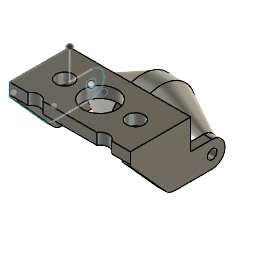
Robot Chassis Version 2 (Autodesk Fusion 360 archive; units mm, degrees)
design "Guide wheel base"
part number: 2026-03-02-16-28-39-596
Autodesk Fusion 360 part; units mm, degrees
sketch "Sketch1" plane through (0, 0, 0) normal (0, 0, 1) x (1, 0, 0)
  line L0 (14.05, 32) -> (-14.05, 32)
  line L1 (-14.05, 32) -> (-14.05, 18)
  line L2 (-14.05, 18) -> (14.05, 18)
  line L3 (14.05, 18) -> (14.05, 32)
  line L4 (14.05, 32) -> (-14.05, 18) construction
  line L5 (-14.05, 32) -> (14.05, 18) construction
  circle A0 centre (0, 25) radius 4
  line L6 (-4, 25) -> (-6.2, 25)
  line L7 (4, 25) -> (6.2, 25)
  circle A1 centre (-8.2, 25) radius 2
  circle A2 centre (8.2, 25) radius 2
  circle A3 centre (-8, 17) radius 2
  circle A4 centre (8, 17) radius 2
  point P0 (0, 25)
  dimension "d1" = 28.1
  dimension "d2" = 14
  dimension "d3" = 8
  dimension "d4" = 2.2
  dimension "d5" = 2.2
  dimension "d6" = 4
  dimension "d7" = 4
  dimension "d8" = 4
  dimension "d9" = 4
  constraint horizontal L0
  constraint perpendicular L0 L1
  constraint parallel L0 L2
  constraint parallel L1 L3
  constraint coincident L4 P0
  constraint coincident L5 P0
  constraint coincident P0 A0.centre
  constraint coincident A0 L6.start
  constraint horizontal L6
  constraint coincident A0 L7.start
  constraint horizontal L7
  constraint coincident L6.end A1
  constraint coincident L7.end A2
  measures "d1" distance of L1.end L2.end
  measures "d2" distance of L0.end L1.end
  measures "d3" diameter of A0
  measures "d4" distance of L6.start L6.end
  measures "d5" distance of L7.start L7.end
  measures "d6" diameter of A1
  measures "d7" diameter of A2
  measures "d8" diameter of A3
  measures "d9" diameter of A4
extrude "Extrude1" add sketch "Sketch1" along normal blind 2 contours L0 L1 L2 L3 A3 A4 makes body 1
move_body "Move1" bodies 1 to x (1, 0, 0) y (0, 1, 0) z (0, 0, 1) at (0, 0, 15)
sketch "Sketch2" plane through (-14.05, 0, 0) normal (-1, 0, 0) x (0, -1, 0)
  line L0 (-32, 15) -> (-18, 15)
  line L1 (-18, 15) -> (-18, 17)
  line L2 (-18, 17) -> (-32, 17)
  line L3 (-32, 17) -> (-32, 15)
  line L4 (-32, 17) -> (-18, 17)
  line L5 (-28.3361, 4) -> (-32, 4)
  line L6 (-32, 4) -> (-37, 4)
  line L7 (-37, 10) -> (-32, 10)
  line L8 (-18.2567, 13.7148) -> (-26.1062, 4.9931)
  arc A0 (-37, 10) -> (-40, 7) centre (-37, 7) ccw
  arc A1 (-40, 7) -> (-37, 4) centre (-37, 7) ccw
  arc A2 (-28.3361, 4) -> (-26.1062, 4.9931) centre (-28.3361, 7) ccw
  line L9 (-18, 17) -> (-18, 14.3837)
  line L10 (-32, 17) -> (-32, 10)
  arc A3 (-18.2567, 13.7148) -> (-18, 14.3837) centre (-19, 14.3837) ccw
  circle A4 centre (-37, 7) radius 1.1
  point P0 (-40, 4)
  dimension "d12" = 13
  dimension "d13" = 8
  dimension "d14" = 6
  dimension "d15" = 3
  dimension "d16" = 3
  dimension "d17" = 3
  dimension "d18" = 1
  dimension "d25" = 2.2
  constraint horizontal L4
  constraint horizontal L5
  constraint coincident L2.end L3.start
  constraint horizontal L6
  constraint horizontal L7
  constraint tangent L7 A0
  constraint coincident P0 L6
  constraint tangent L6 A1
  constraint coincident A0.end A1.start
  constraint tangent L8 A2
  constraint tangent L5 A2
  constraint perpendicular L4 L9
  constraint perpendicular L7 L10
  constraint tangent L8 A3
  constraint tangent L9 A3
  constraint concentric A0 A4
  measures "d12" distance of L2.end L5.end
  measures "d13" distance of L5.end P0
  measures "d14" distance of L5.end L7.end
  measures "d15" radius of A0
  measures "d16" radius of A1
  measures "d17" radius of A2
  measures "d18" radius of A3
  measures "d25" diameter of A4
extrude "Extrude2" add sketch "Sketch2" against normal blind 28.1 contours L0 L5 L6 L7 L8 A0 A1 A2 L9 L10 A3 | A4 bodies 1
sketch "Sketch3" plane through (0, 16.9061, 15.2155) normal (0, -0.743294, -0.668965) x (1, 0, 0)
  line L0 (-14.05, -2.019) -> (-14.05, -13.7528)
  line L1 (-14.05, -13.7528) -> (14.05, -13.7528)
  line L2 (14.05, -13.7528) -> (14.05, -2.019)
  line L3 (14.05, -2.019) -> (-14.05, -2.019)
sketch "Sketch4" plane through (0, 18, 0) normal (0, -1, 0) x (1, 0, 0)
  line L0 (14.05, 14.3837) -> (14.05, 17)
  line L1 (-9.7321, 17) -> (-14.05, 17)
  line L2 (-14.05, 17) -> (-14.05, 14.3837)
  line L3 (-14.05, 14.3837) -> (14.05, 14.3837)
  line L4 (-14.05, 4.9931) -> (-14.05, 4)
  line L5 (-14.05, 4) -> (14.05, 4)
  line L6 (14.05, 4) -> (14.05, 4.9931)
  line L7 (14.05, 4.9931) -> (-14.05, 4.9931)
  line L8 (-14.05, 14.3837) -> (-14.05, 13.7148)
  line L9 (-14.05, 13.7148) -> (14.05, 13.7148)
  line L10 (14.05, 13.7148) -> (14.05, 14.3837)
  line L11 (14.05, 14.3837) -> (-14.05, 14.3837)
  line L12 (-14.05, 13.7148) -> (-14.05, 4.9931)
  line L13 (-14.05, 4.9931) -> (14.05, 4.9931)
  line L14 (14.05, 4.9931) -> (14.05, 13.7148)
  line L15 (14.05, 13.7148) -> (-14.05, 13.7148)
  line L16 (-14.05, 14.3837) -> (-12.05, 14.3837)
  line L17 (-12.05, 14.3837) -> (-12.05, 4)
  line L18 (-12.05, 4) -> (-14.05, 4)
  line L19 (-14.05, 4) -> (-14.05, 14.3837)
  line L20 (14.05, 14.3837) -> (12.05, 14.3837)
  line L21 (12.05, 14.3837) -> (12.05, 4)
  line L22 (12.05, 4) -> (14.05, 4)
  line L23 (14.05, 4) -> (14.05, 14.3837)
  line L24 (-9.7321, 15) -> (-9.7321, 17)
  line L25 (14.05, 17) -> (9.7321, 17)
  line L26 (9.7321, 17) -> (9.7321, 15)
  line L27 (9.7321, 15) -> (6.2679, 15)
  line L28 (6.2679, 15) -> (6.2679, 17)
  line L29 (6.2679, 17) -> (-6.2679, 17)
  line L30 (-6.2679, 17) -> (-6.2679, 15)
  line L31 (-6.2679, 15) -> (-9.7321, 15)
  dimension "d21" = 2
  dimension "d22" = 2
  constraint horizontal L16
  constraint vertical L17
  constraint horizontal L18
  constraint vertical L19
  constraint coincident L5 L17.end
  constraint coincident L2.end L3.start
  constraint horizontal L20
  constraint vertical L21
  constraint horizontal L22
  constraint vertical L23
  constraint coincident L0.start L3.end
  measures "d21" distance of L2.end L16.end
  measures "d22" distance of L0.start L20.end
extrude "Extrude3" cut sketch "Sketch4" against normal blind 25.5 contours L3 L9 L11 L15 L17 L21 | L7 L9 L13 L15 L17 L21 | L5 L7 L13 L17 L21 bodies 1
delete_face "DeleteFace1" 2 faces at (-7.8346, 18.4227, 15) (8.2893, 18.432, 15) on bodies 1
delete_face "DeleteFace2" 3 faces at (-8.0517, 24.35, 15) (1.6687, 25.926, 15) (7.5851, 25.0994, 15) on bodies 1
extrude "Extrude4" cut sketch "Sketch2" against normal blind 33 contours A4 bodies 1
sketch "Sketch5" plane through (0, 0, 0) normal (0, 1, 0) x (1, 0, 0)
  line L0 (12, -7, 37) -> (-12, -7, 37)
  line L1 (-2.2, 1, 37) -> (2.2, 1, 37)
  line L2 (2.2, 1, 37) -> (2.2, -15, 37)
  line L3 (2.2, -15, 37) -> (-2.2, -15, 37)
  line L4 (-2.2, -15, 37) -> (-2.2, 1, 37)
  line L5 (-2.2, 1, 37) -> (2.2, -15, 37) construction
  line L6 (2.2, 1, 37) -> (-2.2, -15, 37) construction
  line L7 (12, -10, 37) -> (12, -4, 37)
  line L8 (12, -4, 37) -> (2.2, 1, 37)
  line L9 (-12, -10, 37) -> (-12, -4, 37)
  line L10 (-12, -4, 37) -> (-2.2, 1, 37)
  line L11 (12, -10, 37) -> (2.2, -15, 37)
  line L12 (-2.2, -15, 37) -> (-12, -10, 37)
  point P0 (0, -7)
  dimension "d28" = 4.4
  dimension "d29" = 16
revolve "Revolve1" add sketch "Sketch5" angle 360 about axis through (12, 37, 7) along (-1, 0, 0) separate body contours L0 L2 L7 L11 | L0 L2 L3 L4 | L0 L4 L9 L12 in plane through (0, 37, 0) normal (0, 1, 0) makes body 2
